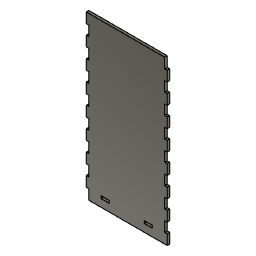
Dice Tower (Back) (Autodesk Fusion 360 design; units mm, degrees)
Autodesk Fusion 360 part; units mm, degrees
sketch "Sketch1" plane through (0, 0, 0) normal (0, 1, 0) x (1, 0, 0)
  line L0 (3.175, -50.8) -> (3.175, -38.1)
  line L1 (3.175, -38.1) -> (3.175, -25.4)
  line L2 (6.35, -12.7) -> (3.175, -12.7)
  line L3 (3.175, -63.5) -> (6.35, -63.5)
  line L4 (3.175, -76.2) -> (3.175, -63.5)
  line L5 (6.35, -25.4) -> (3.175, -25.4)
  line L6 (3.175, -88.9) -> (3.175, -76.2)
  line L7 (6.35, -25.4) -> (6.35, -38.1)
  line L8 (6.35, -38.1) -> (3.175, -38.1)
  line L9 (3.175, -12.7) -> (3.175, 0)
  line L10 (3.175, -60.2676) -> (2.1543, -60.2676)
  line L11 (3.175, 0) -> (3.175, -59.055)
  line L12 (6.35, 0) -> (3.175, 0)
  line L13 (3.175, -25.4) -> (3.175, -12.7)
  line L14 (3.175, -101.6) -> (3.175, -88.9)
  line L15 (3.175, -76.2) -> (6.35, -76.2)
  line L16 (-95.25, -25.4) -> (-95.25, -12.7)
  line L17 (-92.075, -139.7) -> (-95.25, -139.7)
  line L18 (3.175, 0) -> (3.175, -203.2)
  line L19 (-92.075, -50.8) -> (-95.25, -50.8)
  line L20 (3.175, -50.8) -> (6.35, -50.8)
  line L21 (6.35, 0) -> (-4.7498, 0)
  line L22 (3.175, -88.9) -> (6.35, -88.9)
  line L23 (-92.075, -38.1) -> (-92.075, -25.4)
  line L24 (-92.075, -127) -> (-92.075, -114.3)
  line L25 (-95.25, 0) -> (6.35, 0)
  line L26 (-92.075, -203.2) -> (-92.075, -190.5)
  line L27 (3.175, -63.5) -> (3.175, -50.8)
  line L28 (6.35, -50.8) -> (6.35, -63.5)
  line L29 (-92.075, 0) -> (-92.075, -203.2)
  line L30 (6.35, -76.2) -> (6.35, -88.9)
  line L31 (-92.075, -95.25) -> (-92.075, -88.9)
  line L32 (6.35, 0) -> (-5.715, 0)
  line L33 (-95.25, 0) -> (-79.375, 0)
  line L34 (-92.075, -25.4) -> (-95.25, -25.4)
  line L35 (-92.075, -76.2) -> (-92.075, -63.5)
  line L36 (-4.7498, 0) -> (0.3302, 0)
  line L37 (6.35, 0) -> (6.35, -12.7)
  line L38 (6.35, -101.6) -> (3.175, -101.6)
  line L39 (-92.075, -177.8) -> (-95.25, -177.8)
  line L40 (-84.1502, 0) -> (-89.2302, 0)
  line L41 (-92.075, -139.7) -> (-92.075, -127)
  line L42 (-89.5189, -92.8088) -> (-89.7576, -92.8956)
  line L43 (-95.25, -101.6) -> (-95.25, -88.9)
  line L44 (6.35, -177.8) -> (6.35, -190.5)
  line L45 (6.35, -152.4) -> (6.35, -165.1)
  line L46 (3.175, -203.2) -> (3.175, -190.5)
  line L47 (3.175, -190.5) -> (3.175, -177.8)
  line L48 (-92.075, -63.5) -> (-95.25, -63.5)
  line L49 (-92.075, -25.4) -> (-92.075, -12.7)
  line L50 (-92.075, -190.5) -> (-95.25, -190.5)
  line L51 (-92.075, -12.7) -> (-95.25, -12.7)
  line L52 (3.175, -203.2) -> (-95.25, -203.2)
  line L53 (-92.075, -177.8) -> (-92.075, -165.1)
  line L54 (-92.075, -101.6) -> (-92.075, -95.25)
  line L55 (-92.075, -76.2) -> (-95.25, -76.2)
  line L56 (-95.25, -76.2) -> (-95.25, -63.5)
  line L57 (3.175, -114.3) -> (6.35, -114.3)
  line L58 (-95.25, -203.2) -> (-95.25, -190.5)
  line L59 (-92.075, -63.5) -> (-92.075, -50.8)
  line L60 (-92.075, -50.8) -> (-92.075, -38.1)
  line L61 (-92.075, -152.4) -> (-95.25, -152.4)
  line L62 (-92.075, -88.9) -> (-95.25, -88.9)
  line L63 (-92.075, -152.4) -> (-92.075, -139.7)
  line L64 (-95.25, -203.2) -> (-92.075, -203.2)
  line L65 (6.35, -152.4) -> (3.175, -152.4)
  line L66 (-92.075, -165.1) -> (-92.075, -152.4)
  line L67 (-92.075, -203.2) -> (-92.075, -177.8)
  line L68 (-92.075, -165.1) -> (-95.25, -165.1)
  line L69 (-92.075, -114.3) -> (-95.25, -114.3)
  line L70 (6.35, -101.6) -> (6.35, -114.3)
  line L71 (-95.25, -127) -> (-95.25, -114.3)
  line L72 (-92.075, -114.3) -> (-92.075, -101.6)
  line L73 (6.35, -139.7) -> (6.35, -127)
  line L74 (6.35, -127) -> (6.35, -139.7)
  line L75 (3.175, -177.8) -> (6.35, -177.8)
  line L76 (3.175, -165.1) -> (6.35, -165.1)
  line L77 (-92.075, -38.1) -> (-95.25, -38.1)
  line L78 (6.35, -114.3) -> (6.35, -101.6)
  line L79 (-95.25, 0) -> (-84.1502, 0)
  line L80 (-92.075, -127) -> (-95.25, -127)
  line L81 (3.175, -152.4) -> (3.175, -139.7)
  line L82 (-95.25, -177.8) -> (-95.25, -165.1)
  line L83 (6.35, -165.1) -> (6.35, -152.4)
  line L84 (-92.075, -101.6) -> (-95.25, -101.6)
  line L85 (3.175, -139.7) -> (6.35, -139.7)
  line L86 (-95.25, 0) -> (-92.075, 0)
  line L87 (-95.25, -152.4) -> (-95.25, -139.7)
  line L88 (3.175, -127) -> (3.175, -114.3)
  line L89 (6.35, -127) -> (3.175, -127)
  line L90 (3.175, -190.5) -> (6.35, -190.5)
  line L91 (-92.075, -88.9) -> (-92.075, -76.2)
  line L92 (-95.25, 0) -> (-93.6625, 0)
  line L93 (-92.075, -190.5) -> (-92.075, -177.8)
  line L94 (3.175, -177.8) -> (3.175, -165.1)
  line L95 (-95.25, -50.8) -> (-95.25, -38.1)
  point P0 (6.35, 0)
  point P1 (6.35, 0)
  dimension "d9" = 11.0998
  dimension "d10" = 11.0998
  dimension "d14" = 5.08
  dimension "d15" = 5.08
  dimension "d27" = 3.175
  dimension "d28" = 3.175
  dimension "d40" = 3.175
  dimension "d41" = 3.175
  dimension "d42" = 12.7
  dimension "d43" = 12.7
  dimension "d44" = 12.7
  dimension "d45" = 12.7
  dimension "d46" = 12.7
  dimension "d47" = 12.7
  dimension "d48" = 12.7
  dimension "d49" = 12.7
  dimension "d50" = 6.35
  dimension "d52" = 12.7
  dimension "d53" = 12.7
  dimension "d54" = 12.7
  dimension "d55" = 12.7
  dimension "d56" = 12.7
  dimension "d57" = 12.7
  constraint coincident P1 P0
  constraint perpendicular L37 L52
  constraint perpendicular L52 L58
  constraint perpendicular L25 L37
  constraint perpendicular L32 L37
  constraint perpendicular L33 L58
  constraint perpendicular L58 L92
  constraint coincident L40.start L25
  constraint perpendicular L21 L37
  constraint perpendicular L37 L90
  constraint perpendicular L47 L90
  constraint coincident L44.start L37
  constraint perpendicular L37 L75
  constraint perpendicular L75 L94
  constraint perpendicular L37 L76
  constraint collinear L37 L44
  constraint perpendicular L76 L83
  constraint perpendicular L65 L83
  constraint parallel L12 L32
  constraint perpendicular L18 L52
  constraint perpendicular L65 L81
  constraint coincident L88.start L18
  constraint perpendicular L18 L89
  constraint perpendicular L88 L89
  constraint perpendicular L57 L88
  constraint perpendicular L18 L38
  constraint perpendicular L14 L38
  constraint parallel L0 L1
  constraint parallel L13 L18
  constraint coincident L15.end L37
  constraint coincident L20.end L37
  constraint coincident L5.start L37
  constraint collinear L37 L45
  constraint collinear L37 L74
  constraint collinear L37 L70
  constraint collinear L30 L37
  constraint collinear L28 L37
  constraint collinear L7 L37
  constraint perpendicular L58 L64
  constraint perpendicular L58 L86
  constraint perpendicular L26 L52
  constraint perpendicular L50 L58
  constraint perpendicular L50 L93
  constraint coincident L39.end L58
  constraint perpendicular L39 L58
  constraint perpendicular L39 L53
  constraint coincident L68.end L58
  constraint perpendicular L58 L68
  constraint perpendicular L66 L68
  constraint coincident L61.end L58
  constraint perpendicular L58 L61
  constraint perpendicular L61 L63
  constraint coincident L17.end L58
  constraint perpendicular L17 L58
  constraint perpendicular L17 L41
  constraint coincident L71.start L58
  constraint perpendicular L58 L80
  constraint perpendicular L24 L80
  constraint coincident L69.end L58
  constraint perpendicular L58 L69
  constraint perpendicular L69 L72
  constraint perpendicular L58 L84
  constraint perpendicular L54 L84
  constraint parallel L29 L31
  constraint coincident L43.end L58
  constraint perpendicular L58 L62
  constraint perpendicular L62 L91
  constraint coincident L55.end L58
  constraint perpendicular L55 L58
  constraint perpendicular L35 L55
  constraint coincident L48.end L58
  constraint perpendicular L48 L58
  constraint perpendicular L48 L59
  constraint coincident L19.end L58
  constraint perpendicular L19 L58
  constraint perpendicular L19 L60
  constraint coincident L77.end L58
  constraint perpendicular L58 L77
  constraint perpendicular L23 L77
  constraint perpendicular L23 L34
  constraint perpendicular L34 L49
  constraint perpendicular L49 L51
  constraint collinear L58 L82
  constraint coincident L43.start L58
  constraint collinear L82 L87
  constraint collinear L71 L87
  constraint collinear L43 L71
  constraint collinear L43 L56
  constraint collinear L56 L95
  constraint collinear L16 L95
  constraint coincident L11.end L27
  constraint coincident L10.start L27
  measures "d9" distance of L40.start L25.start
  measures "d10" distance of P1 L21.end
  measures "d14" distance of L36.end L21.end
  measures "d15" distance of L40.start L40.end
  measures "d27" distance of L65.end L45.start
  measures "d28" distance of P1 L9.end
  measures "d40" distance of L52.end L26.start
  measures "d41" distance of L25.start L29.start
  measures "d42" distance of L26.end L26.start
  measures "d43" distance of L39.start L26.end
  measures "d44" distance of L39.start L53.end
  measures "d45" distance of L61.start L53.end
  measures "d46" distance of L61.start L17.start
  measures "d47" distance of L24.start L17.start
  measures "d48" distance of L24.start L24.end
  measures "d49" distance of L54.start L24.end
  measures "d50" distance of L54.start L31.start
  measures "d52" distance of L35.start L31.end
  measures "d53" distance of L35.start L35.end
  measures "d54" distance of L19.start L35.end
  measures "d55" distance of L23.start L19.start
  measures "d56" distance of L23.end L23.start
  measures "d57" distance of L49.end L23.end
extrude "Extrude1" add sketch "Sketch1" along normal blind 3.175
sketch "Sketch2" plane through (0, 0, 0) normal (0, -1, 0) x (1, 0, 0)
  line L0 (-95.25, 63.5) -> (-92.075, 63.5)
  line L1 (-92.075, 63.5) -> (-92.075, 50.8)
  line L2 (-92.075, 50.8) -> (-95.25, 50.8)
  line L3 (-95.25, 50.8) -> (-95.25, 38.1)
  line L4 (-95.25, 38.1) -> (-92.075, 38.1)
  line L5 (-92.075, 38.1) -> (-92.075, 25.4)
  line L6 (-92.075, 25.4) -> (-95.25, 25.4)
  line L7 (-95.25, 25.4) -> (-95.25, 12.7)
  line L8 (-95.25, 12.7) -> (-92.075, 12.7)
  line L9 (-92.075, 12.7) -> (-92.075, 0)
  line L10 (-92.075, 0) -> (6.35, 0)
  line L11 (6.35, 0) -> (6.35, 12.7)
  line L12 (6.35, 12.7) -> (3.175, 12.7)
  line L13 (3.175, 12.7) -> (3.175, 25.4)
  line L14 (3.175, 25.4) -> (6.35, 25.4)
  line L15 (6.35, 25.4) -> (6.35, 38.1)
  line L16 (6.35, 38.1) -> (3.175, 38.1)
  line L17 (3.175, 38.1) -> (3.175, 50.8)
  line L18 (3.175, 50.8) -> (6.35, 50.8)
  line L19 (6.35, 50.8) -> (6.35, 63.5)
  line L20 (6.35, 63.5) -> (3.175, 63.5)
  line L21 (3.175, 63.5) -> (3.175, 76.2)
  line L22 (3.175, 76.2) -> (6.35, 76.2)
  line L23 (6.35, 76.2) -> (6.35, 88.9)
  line L24 (6.35, 88.9) -> (3.175, 88.9)
  line L25 (3.175, 88.9) -> (3.175, 101.6)
  line L26 (3.175, 101.6) -> (6.35, 101.6)
  line L27 (6.35, 101.6) -> (6.35, 114.3)
  line L28 (6.35, 114.3) -> (3.175, 114.3)
  line L29 (3.175, 114.3) -> (3.175, 127)
  line L30 (3.175, 127) -> (6.35, 127)
  line L31 (6.35, 127) -> (6.35, 139.7)
  line L32 (6.35, 139.7) -> (3.175, 139.7)
  line L33 (3.175, 139.7) -> (3.175, 152.4)
  line L34 (3.175, 152.4) -> (6.35, 152.4)
  line L35 (6.35, 152.4) -> (6.35, 165.1)
  line L36 (6.35, 165.1) -> (3.175, 165.1)
  line L37 (3.175, 165.1) -> (3.175, 177.8)
  line L38 (3.175, 177.8) -> (6.35, 177.8)
  line L39 (6.35, 177.8) -> (6.35, 190.5)
  line L40 (6.35, 190.5) -> (3.175, 190.5)
  line L41 (3.175, 190.5) -> (3.175, 203.2)
  line L42 (3.175, 203.2) -> (-95.25, 203.2)
  line L43 (-95.25, 203.2) -> (-95.25, 190.5)
  line L44 (-95.25, 190.5) -> (-92.075, 190.5)
  line L45 (-92.075, 190.5) -> (-92.075, 177.8)
  line L46 (-92.075, 177.8) -> (-95.25, 177.8)
  line L47 (-95.25, 177.8) -> (-95.25, 165.1)
  line L48 (-95.25, 165.1) -> (-92.075, 165.1)
  line L49 (-92.075, 165.1) -> (-92.075, 152.4)
  line L50 (-92.075, 152.4) -> (-95.25, 152.4)
  line L51 (-95.25, 152.4) -> (-95.25, 139.7)
  line L52 (-95.25, 139.7) -> (-92.075, 139.7)
  line L53 (-92.075, 139.7) -> (-92.075, 127)
  line L54 (-92.075, 127) -> (-95.25, 127)
  line L55 (-95.25, 127) -> (-95.25, 114.3)
  line L56 (-95.25, 114.3) -> (-92.075, 114.3)
  line L57 (-92.075, 114.3) -> (-92.075, 101.6)
  line L58 (-92.075, 101.6) -> (-95.25, 101.6)
  line L59 (-95.25, 101.6) -> (-95.25, 88.9)
  line L60 (-95.25, 88.9) -> (-92.075, 88.9)
  line L61 (-92.075, 88.9) -> (-92.075, 76.2)
  line L62 (-92.075, 76.2) -> (-95.25, 76.2)
  line L63 (-95.25, 76.2) -> (-95.25, 63.5)
  line L64 (6.35, 0) -> (-12.3698, 0)
  line L65 (-12.3698, 0) -> (-12.3698, 9.525)
  line L66 (-92.075, 0) -> (-76.5302, 0)
  line L67 (-76.5302, 0) -> (-76.5302, 9.525)
  line L68 (-76.5302, 9.525) -> (-66.3702, 9.525)
  line L69 (-66.3702, 9.525) -> (-66.3702, 12.7)
  line L70 (-66.3702, 12.7) -> (-76.5302, 12.7)
  line L71 (-76.5302, 12.7) -> (-76.5302, 9.525)
  line L72 (-12.3698, 9.525) -> (-22.5298, 9.525)
  line L73 (-22.5298, 9.525) -> (-22.5298, 12.7)
  line L74 (-22.5298, 12.7) -> (-12.3698, 12.7)
  line L75 (-12.3698, 12.7) -> (-12.3698, 9.525)
  dimension "d105" = 18.7198
  dimension "d106" = 9.525
  dimension "d107" = 15.5448
  dimension "d108" = 9.525
  dimension "d109" = 10.16
  dimension "d110" = 3.175
  dimension "d111" = 10.16
  dimension "d112" = 10.16
  dimension "d113" = 10.16
  constraint coincident L10.end L11.start
  constraint perpendicular L11 L64
  constraint perpendicular L64 L65
  constraint coincident L9.end L10.start
  constraint perpendicular L9 L66
  constraint perpendicular L66 L67
  constraint perpendicular L67 L68
  constraint perpendicular L68 L69
  constraint perpendicular L69 L70
  constraint perpendicular L65 L72
  constraint perpendicular L72 L73
  constraint perpendicular L73 L74
  measures "d105" distance of L10.end L64.end
  measures "d106" distance of L64.end L65.end
  measures "d107" distance of L9.end L66.end
  measures "d108" distance of L66.end L67.end
  measures "d109" distance of L67.end L68.end
  measures "d110" distance of L68.end L69.end
  measures "d111" distance of L69.end L70.end
  measures "d112" distance of L65.end L72.end
  measures "d113" distance of L73.end L74.end
extrude "Extrude2" cut sketch "Sketch2" against normal blind 20.32 contours L68 L69 L70 L71 | L72 L73 L74 L75
equation "d9 = 0.5 in - 0.063 in"
